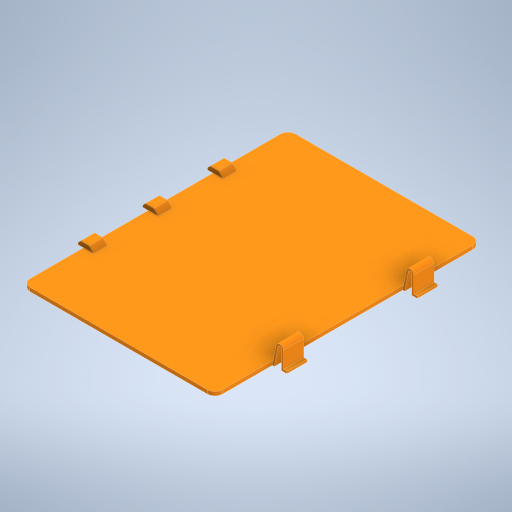
# Autodesk Inventor part: Toolbox cover
Saved by Autodesk Inventor 2023 (Build 270158000, 158)
## iProperties
Created: 2023-03-08
Part Number: Toolbox cover
Material: Типовые
Document SubType Name: Modeling
Designer: Josh
Density: 1 g/cm^3
Appearance: Оранжевый
Author: Josh
Autodesk Inventor part; units mm, degrees
ref_plane "YZ Plane" through (0, 0, 0) normal (1, 0, 0) x (0, 1, 0)
sketch "Эскиз1" plane through (0, 0, 0) normal (0, 1, 0) x (-1, 0, 0)
  line L0 (-48, -71.75) -> (48, -71.75)
  line L1 (52, -67.75) -> (52, 67.75)
  line L2 (48, 71.75) -> (-48, 71.75)
  line L3 (-52, 67.75) -> (-52, -67.75)
  line L4 (-52, -71.75) -> (52, 71.75) construction
  line L5 (52, -71.75) -> (-52, 71.75) construction
  arc A0 (52, 67.75) -> (48, 71.75) centre (48, 67.75) ccw
  arc A1 (48, -71.75) -> (52, -67.75) centre (48, -67.75) ccw
  arc A2 (-52, -67.75) -> (-48, -71.75) centre (-48, -67.75) ccw
  arc A3 (-48, 71.75) -> (-52, 67.75) centre (-48, 67.75) ccw
  line L6 (-52, 40.75) -> (-54, 40.75)
  line L7 (-54, 40.75) -> (-54, 29.75)
  line L8 (-54, 29.75) -> (-52, 29.75)
  line L9 (-52, 29.75) -> (-52, 40.75)
  line L10 (-52, 0) -> (52, 0)
  line L11 (-52, -40.75) -> (-54, -40.75)
  line L12 (-54, -40.75) -> (-54, -29.75)
  line L13 (-54, -29.75) -> (-52, -29.75)
  line L14 (-52, -29.75) -> (-52, -40.75)
  circle A4 centre (-30, -63.75) radius 2.05
  line L15 (0, -71.75) -> (0, 71.75)
  circle A5 centre (30, -63.75) radius 2.05
  circle A6 centre (-30, 63.75) radius 2.05
  circle A7 centre (30, 63.75) radius 2.05
  point P0 (0, 0)
  point P1 (-52, 29.75)
  point P2 (-52, -29.75)
  point P3 (-52, -40.75)
  dimension "d0" = 104
  dimension "d1" = 143.5
  dimension "d2" = 4
  dimension "d3" = 2
  dimension "d4" = 11
  dimension "d5" = 31
  dimension "d6" = 4.1
  dimension "d7" = 8
  dimension "d8" = 60
  constraints: 32 end point, 9 point on line, 8 centre point, 8 point on circle, 8 tangent, 7 symmetric about line, 6 midpoint, 4 parallel, 3 equal radius, 2 horizontal, 2 perpendicular, 3 other
  measures "d0" distance of L5.end L4.end
  measures "d1" distance of L4.end L5.start
  measures "d2" radius of A0
  measures "d3" distance of L8.end L7.end
  measures "d4" distance of L7.end L6.end
  measures "d5" distance between parallel lines of L2 L6
  measures "d6" diameter of A4
  measures "d7" distance from line of L0 A4.centre
  measures "d8" distance of A5.centre A4.centre
extrude "Выдавливание1" add sketch "Эскиз1" along normal blind 2 contours A2 L3 L10 L15 L0 | L15 L10 L1 A1 L0 | L15 L2 A0 L1 L10 | L10 L3 A3 L2 L15 | A4 | A5 | A6 | A7
ref_plane "РабПлоскость1" through (-48, 0, 40.75) normal (0, 0, 1) x (1, 0, 0)
sketch "Эскиз3" plane through (-48, 0, 40.75) normal (0, 0, 1) x (1, 0, 0)
  line L0 (100, 0) -> (102.0373, 10.3941)
  arc A0 (106, 10.0094) -> (102.0373, 10.3941) centre (104, 10.0094) ccw
  line L1 (100, 2) -> (96, 2) projected
  line L2 (106, 10.0094) -> (106, 1.1)
  line L3 (101.1209, 0) -> (103.1168, 10.1825)
  arc A1 (104.9, 10.0094) -> (103.1168, 10.1825) centre (104, 10.0094) ccw
  line L4 (104.9, 10.0094) -> (104.9, 0)
  line L5 (100, 0) -> (96, 0) projected
  line L6 (100, 0) -> (101.1209, 0)
  line L7 (104.9, 0) -> (109, 0)
  line L8 (104.9, 0) -> (107.9, 0)
  line L9 (107.9, 0) -> (107.9, 1.1)
  line L10 (107.9, 1.1) -> (106, 1.1)
  line L11 (104.9, 1.1) -> (104.9, 0)
  line L12 (100, 2) -> (100.392, 2)
  line L13 (100, 2) -> (100, 0)
  point P0 (48, 0)
  point P1 (104.1933, 12)
  dimension "d19" = 10
  dimension "d20" = 2
  dimension "d21" = 6
  dimension "d22" = 1.1
  dimension "d23" = 1.1
  dimension "d24" = 1.1
  dimension "d25" = 3
  constraints: 24 end point, 5 point on circle, 3 horizontal, 3 tangent, 2 centre point, 2 parallel, 2 perpendicular, 1 collinear, 1 horizontal alignment, 1 point on line, 1 vertical
  measures "d19" vertical distance of point (104.193, 12) L1.start
  measures "d20" radius of A0
  measures "d21" distance from line of L1.start L2
  measures "d22" distance between parallel lines of L0 L3
  measures "d23" radial gap between concentric circles of A0 A1
  measures "d24" distance between parallel lines of L7 L10
  measures "d25" distance between parallel lines of L4 L9
extrude "Выдавливание2" add sketch "Эскиз3" against normal blind 11
mirror "Зеркальное отражение1" about plane through (0, 0, 0) normal (0, 0, 1) of "Выдавливание2"
sketch "Эскиз4" plane through (0, 2, 0) normal (0, 1, 0) x (1, 0, 0)
  line L0 (-46.5, -31.25) -> (-55, -31.25)
  line L1 (-55, -31.25) -> (-55, -38.75)
  line L2 (-55, -38.75) -> (-46.5, -38.75)
  line L3 (-46.5, -38.75) -> (-46.5, -31.25)
  line L4 (-52, 67.75) -> (-52, -67.75) projected
  line L5 (-48, -71.75) -> (48, -71.75) projected
  point P0 (0, 0)
  dimension "d28" = 7.5
  dimension "d29" = 3
  dimension "d30" = 33
  dimension "d31" = 5.5
  constraints: 8 end point, 2 parallel, 1 horizontal, 1 perpendicular
  measures "d28" distance between parallel lines of L2 L0
  measures "d29" distance between parallel lines of L1 L4
  measures "d30" distance between parallel lines of L5 L2
  measures "d31" distance between parallel lines of L3 L4
extrude "Выдавливание3" add sketch "Эскиз4" along normal blind 2.5
mirror "Зеркальное отражение2" about plane through (0, 0, 0) normal (0, 0, 1) of "Выдавливание3"
ref_plane "РабПлоскость3" through (-55, 2, 17.5) normal (0, 0, 1) x (1, 0, 0)
ref_plane "РабПлоскость2" through (-55, 2, 35) normal (0, 0, 1) x (1, 0, 0)
mirror "Зеркальное отражение3" about plane through (-55, 2, 17.5) normal (0, 0, 1) of "Выдавливание3"
chamfer "Фаска1" distance 1.5 angle 45 3 edges at (-55, 4.5, 35) (-55, 4.5, 0) (-55, 4.5, -35)
chamfer "Фаска2" distance 2.5 angle 45 3 edges at (-46.5, 4.5, 35) (-46.5, 4.5, -35) (-46.5, 4.5, 0)
